Autodesk Inventor part; units mm, degrees
(part 3 of 3)
  line L1419 (-51.1011, -48.3705) -> (-50.3814, -49.0902) construction
  line L1420 (-50.3814, -49.0902) -> (-50.3814, -49.9795) construction
  spline S136 degree 3 poles (-46.3996, -18.0009) (-46.3996, -18.8902) (-47.1193, -19.6113) (-48.0086, -19.6113) knots 0 0 0 0 1 1 1 1
  line L1421 (-46.3996, -18.0009) -> (-46.3996, -18.8902) construction
  line L1422 (-46.3996, -18.8902) -> (-47.1193, -19.6113) construction
  line L1423 (-47.1193, -19.6113) -> (-48.0086, -19.6113) construction
  spline S137 degree 3 poles (-48.0086, -19.6113) (-48.8993, -19.6113) (-49.619, -18.8902) (-49.619, -18.0009) knots 0 0 0 0 1 1 1 1
  line L1424 (-48.0086, -19.6113) -> (-48.8993, -19.6113) construction
  line L1425 (-48.8993, -19.6113) -> (-49.619, -18.8902) construction
  line L1426 (-49.619, -18.8902) -> (-49.619, -18.0009) construction
  spline S138 degree 3 poles (-49.619, -18.0009) (-49.619, -17.1116) (-48.8993, -16.3919) (-48.0086, -16.3919) knots 0 0 0 0 1 1 1 1
  line L1427 (-49.619, -18.0009) -> (-49.619, -17.1116) construction
  line L1428 (-49.619, -17.1116) -> (-48.8993, -16.3919) construction
  line L1429 (-48.8993, -16.3919) -> (-48.0086, -16.3919) construction
  spline S139 degree 3 poles (-48.0086, -16.3919) (-47.1193, -16.3919) (-46.3996, -17.1116) (-46.3996, -18.0009) knots 0 0 0 0 1 1 1 1
  line L1430 (-48.0086, -16.3919) -> (-47.1193, -16.3919) construction
  line L1431 (-47.1193, -16.3919) -> (-46.3996, -17.1116) construction
  line L1432 (-46.3996, -17.1116) -> (-46.3996, -18.0009) construction
  spline S140 degree 3 poles (-72.7019, -7.3708) (-72.7019, -8.0905) (-73.2534, -8.6406) (-73.9731, -8.6406) knots 0 0 0 0 1 1 1 1
  line L1433 (-72.7019, -7.3708) -> (-72.7019, -8.0905) construction
  line L1434 (-72.7019, -8.0905) -> (-73.2534, -8.6406) construction
  line L1435 (-73.2534, -8.6406) -> (-73.9731, -8.6406) construction
  spline S141 degree 3 poles (-73.9731, -8.6406) (-74.6928, -8.6406) (-75.2429, -8.0905) (-75.2429, -7.3708) knots 0 0 0 0 1 1 1 1
  line L1436 (-73.9731, -8.6406) -> (-74.6928, -8.6406) construction
  line L1437 (-74.6928, -8.6406) -> (-75.2429, -8.0905) construction
  line L1438 (-75.2429, -8.0905) -> (-75.2429, -7.3708) construction
  spline S142 degree 3 poles (-75.2429, -7.3708) (-75.2429, -6.6497) (-74.6928, -6.0996) (-73.9731, -6.0996) knots 0 0 0 0 1 1 1 1
  line L1439 (-75.2429, -7.3708) -> (-75.2429, -6.6497) construction
  line L1440 (-75.2429, -6.6497) -> (-74.6928, -6.0996) construction
  line L1441 (-74.6928, -6.0996) -> (-73.9731, -6.0996) construction
  spline S143 degree 3 poles (-73.9731, -6.0996) (-73.2534, -6.0996) (-72.7019, -6.6497) (-72.7019, -7.3708) knots 0 0 0 0 1 1 1 1
  line L1442 (-73.9731, -6.0996) -> (-73.2534, -6.0996) construction
  line L1443 (-73.2534, -6.0996) -> (-72.7019, -6.6497) construction
  line L1444 (-72.7019, -6.6497) -> (-72.7019, -7.3708) construction
  spline S144 degree 3 poles (-72.7019, 7.3694) (-72.7019, 6.6497) (-73.2534, 6.0982) (-73.9731, 6.0982) knots 0 0 0 0 1 1 1 1
  line L1445 (-72.7019, 7.3694) -> (-72.7019, 6.6497) construction
  line L1446 (-72.7019, 6.6497) -> (-73.2534, 6.0982) construction
  line L1447 (-73.2534, 6.0982) -> (-73.9731, 6.0982) construction
  spline S145 degree 3 poles (-73.9731, 6.0982) (-74.6928, 6.0982) (-75.2429, 6.6497) (-75.2429, 7.3694) knots 0 0 0 0 1 1 1 1
  line L1448 (-73.9731, 6.0982) -> (-74.6928, 6.0982) construction
  line L1449 (-74.6928, 6.0982) -> (-75.2429, 6.6497) construction
  line L1450 (-75.2429, 6.6497) -> (-75.2429, 7.3694) construction
  spline S146 degree 3 poles (-75.2429, 7.3694) (-75.2429, 8.0891) (-74.6928, 8.6406) (-73.9731, 8.6406) knots 0 0 0 0 1 1 1 1
  line L1451 (-75.2429, 7.3694) -> (-75.2429, 8.0891) construction
  line L1452 (-75.2429, 8.0891) -> (-74.6928, 8.6406) construction
  line L1453 (-74.6928, 8.6406) -> (-73.9731, 8.6406) construction
  spline S147 degree 3 poles (-73.9731, 8.6406) (-73.2534, 8.6406) (-72.7019, 8.0891) (-72.7019, 7.3694) knots 0 0 0 0 1 1 1 1
  line L1454 (-73.9731, 8.6406) -> (-73.2534, 8.6406) construction
  line L1455 (-73.2534, 8.6406) -> (-72.7019, 8.0891) construction
  line L1456 (-72.7019, 8.0891) -> (-72.7019, 7.3694) construction
  spline S148 degree 3 poles (-46.3996, 18.0009) (-46.3996, 17.1116) (-47.1193, 16.3905) (-48.0086, 16.3905) knots 0 0 0 0 1 1 1 1
  line L1457 (-46.3996, 18.0009) -> (-46.3996, 17.1116) construction
  line L1458 (-46.3996, 17.1116) -> (-47.1193, 16.3905) construction
  line L1459 (-47.1193, 16.3905) -> (-48.0086, 16.3905) construction
  spline S149 degree 3 poles (-48.0086, 16.3905) (-48.8993, 16.3905) (-49.619, 17.1116) (-49.619, 18.0009) knots 0 0 0 0 1 1 1 1
  line L1460 (-48.0086, 16.3905) -> (-48.8993, 16.3905) construction
  line L1461 (-48.8993, 16.3905) -> (-49.619, 17.1116) construction
  line L1462 (-49.619, 17.1116) -> (-49.619, 18.0009) construction
  spline S150 degree 3 poles (-49.619, 18.0009) (-49.619, 18.8902) (-48.8993, 19.6099) (-48.0086, 19.6099) knots 0 0 0 0 1 1 1 1
  line L1463 (-49.619, 18.0009) -> (-49.619, 18.8902) construction
  line L1464 (-49.619, 18.8902) -> (-48.8993, 19.6099) construction
  line L1465 (-48.8993, 19.6099) -> (-48.0086, 19.6099) construction
  spline S151 degree 3 poles (-48.0086, 19.6099) (-47.1193, 19.6099) (-46.3996, 18.8902) (-46.3996, 18.0009) knots 0 0 0 0 1 1 1 1
  line L1466 (-48.0086, 19.6099) -> (-47.1193, 19.6099) construction
  line L1467 (-47.1193, 19.6099) -> (-46.3996, 18.8902) construction
  line L1468 (-46.3996, 18.8902) -> (-46.3996, 18.0009) construction
  spline S152 degree 3 poles (-50.3814, 50.0209) (-50.3814, 49.1316) (-51.1011, 48.4119) (-51.9904, 48.4119) knots 0 0 0 0 1 1 1 1
  line L1469 (-50.3814, 50.0209) -> (-50.3814, 49.1316) construction
  line L1470 (-50.3814, 49.1316) -> (-51.1011, 48.4119) construction
  line L1471 (-51.1011, 48.4119) -> (-51.9904, 48.4119) construction
  spline S153 degree 3 poles (-51.9904, 48.4119) (-52.8797, 48.4119) (-53.6008, 49.1316) (-53.6008, 50.0209) knots 0 0 0 0 1 1 1 1
  line L1472 (-51.9904, 48.4119) -> (-52.8797, 48.4119) construction
  line L1473 (-52.8797, 48.4119) -> (-53.6008, 49.1316) construction
  line L1474 (-53.6008, 49.1316) -> (-53.6008, 50.0209) construction
  spline S154 degree 3 poles (-53.6008, 50.0209) (-53.6008, 50.9102) (-52.8797, 51.6299) (-51.9904, 51.6299) knots 0 0 0 0 1 1 1 1
  line L1475 (-53.6008, 50.0209) -> (-53.6008, 50.9102) construction
  line L1476 (-53.6008, 50.9102) -> (-52.8797, 51.6299) construction
  line L1477 (-52.8797, 51.6299) -> (-51.9904, 51.6299) construction
  spline S155 degree 3 poles (-51.9904, 51.6299) (-51.1011, 51.6299) (-50.3814, 50.9102) (-50.3814, 50.0209) knots 0 0 0 0 1 1 1 1
  line L1478 (-51.9904, 51.6299) -> (-51.1011, 51.6299) construction
  line L1479 (-51.1011, 51.6299) -> (-50.3814, 50.9102) construction
  line L1480 (-50.3814, 50.9102) -> (-50.3814, 50.0209) construction
  spline S156 degree 3 poles (-7.7299, 44.0068) (-7.7299, 43.2871) (-8.2801, 42.7356) (-8.9998, 42.7356) knots 0 0 0 0 1 1 1 1
  line L1481 (-7.7299, 44.0068) -> (-7.7299, 43.2871) construction
  line L1482 (-7.7299, 43.2871) -> (-8.2801, 42.7356) construction
  line L1483 (-8.2801, 42.7356) -> (-8.9998, 42.7356) construction
  spline S157 degree 3 poles (-8.9998, 42.7356) (-9.7208, 42.7356) (-10.271, 43.2871) (-10.271, 44.0068) knots 0 0 0 0 1 1 1 1
  line L1484 (-8.9998, 42.7356) -> (-9.7208, 42.7356) construction
  line L1485 (-9.7208, 42.7356) -> (-10.271, 43.2871) construction
  line L1486 (-10.271, 43.2871) -> (-10.271, 44.0068) construction
  spline S158 degree 3 poles (-10.271, 44.0068) (-10.271, 44.7265) (-9.7208, 45.2766) (-8.9998, 45.2766) knots 0 0 0 0 1 1 1 1
  line L1487 (-10.271, 44.0068) -> (-10.271, 44.7265) construction
  line L1488 (-10.271, 44.7265) -> (-9.7208, 45.2766) construction
  line L1489 (-9.7208, 45.2766) -> (-8.9998, 45.2766) construction
  spline S159 degree 3 poles (-8.9998, 45.2766) (-8.2801, 45.2766) (-7.7299, 44.7265) (-7.7299, 44.0068) knots 0 0 0 0 1 1 1 1
  line L1490 (-8.9998, 45.2766) -> (-8.2801, 45.2766) construction
  line L1491 (-8.2801, 45.2766) -> (-7.7299, 44.7265) construction
  line L1492 (-7.7299, 44.7265) -> (-7.7299, 44.0068) construction
  spline S160 degree 3 poles (52.626, 50.0209) (52.626, 49.1316) (51.9063, 48.4119) (51.017, 48.4119) knots 0 0 0 0 1 1 1 1
  line L1493 (52.626, 50.0209) -> (52.626, 49.1316) construction
  line L1494 (52.626, 49.1316) -> (51.9063, 48.4119) construction
  line L1495 (51.9063, 48.4119) -> (51.017, 48.4119) construction
  spline S161 degree 3 poles (51.017, 48.4119) (50.1277, 48.4119) (49.408, 49.1316) (49.408, 50.0209) knots 0 0 0 0 1 1 1 1
  line L1496 (51.017, 48.4119) -> (50.1277, 48.4119) construction
  line L1497 (50.1277, 48.4119) -> (49.408, 49.1316) construction
  line L1498 (49.408, 49.1316) -> (49.408, 50.0209) construction
  spline S162 degree 3 poles (49.408, 50.0209) (49.408, 50.9102) (50.1277, 51.6299) (51.017, 51.6299) knots 0 0 0 0 1 1 1 1
  line L1499 (49.408, 50.0209) -> (49.408, 50.9102) construction
  line L1500 (49.408, 50.9102) -> (50.1277, 51.6299) construction
  line L1501 (50.1277, 51.6299) -> (51.017, 51.6299) construction
  spline S163 degree 3 poles (51.017, 51.6299) (51.9063, 51.6299) (52.626, 50.9102) (52.626, 50.0209) knots 0 0 0 0 1 1 1 1
  line L1502 (51.017, 51.6299) -> (51.9063, 51.6299) construction
  line L1503 (51.9063, 51.6299) -> (52.626, 50.9102) construction
  line L1504 (52.626, 50.9102) -> (52.626, 50.0209) construction
  spline S164 degree 3 poles (10.271, 44.0068) (10.271, 43.2871) (9.7208, 42.7356) (9.0011, 42.7356) knots 0 0 0 0 1 1 1 1
  line L1505 (10.271, 44.0068) -> (10.271, 43.2871) construction
  line L1506 (10.271, 43.2871) -> (9.7208, 42.7356) construction
  line L1507 (9.7208, 42.7356) -> (9.0011, 42.7356) construction
  spline S165 degree 3 poles (9.0011, 42.7356) (8.28, 42.7356) (7.7299, 43.2871) (7.7299, 44.0068) knots 0 0 0 0 1 1 1 1
  line L1508 (9.0011, 42.7356) -> (8.28, 42.7356) construction
  line L1509 (8.28, 42.7356) -> (7.7299, 43.2871) construction
  line L1510 (7.7299, 43.2871) -> (7.7299, 44.0068) construction
  spline S166 degree 3 poles (7.7299, 44.0068) (7.7299, 44.7265) (8.28, 45.2766) (9.0011, 45.2766) knots 0 0 0 0 1 1 1 1
  line L1511 (7.7299, 44.0068) -> (7.7299, 44.7265) construction
  line L1512 (7.7299, 44.7265) -> (8.28, 45.2766) construction
  line L1513 (8.28, 45.2766) -> (9.0011, 45.2766) construction
  spline S167 degree 3 poles (9.0011, 45.2766) (9.7208, 45.2766) (10.271, 44.7265) (10.271, 44.0068) knots 0 0 0 0 1 1 1 1
  line L1514 (9.0011, 45.2766) -> (9.7208, 45.2766) construction
  line L1515 (9.7208, 45.2766) -> (10.271, 44.7265) construction
  line L1516 (10.271, 44.7265) -> (10.271, 44.0068) construction
  spline S168 degree 3 poles (20.606, 18.0009) (20.606, 17.1116) (19.8863, 16.3905) (18.997, 16.3905) knots 0 0 0 0 1 1 1 1
  line L1517 (20.606, 18.0009) -> (20.606, 17.1116) construction
  line L1518 (20.606, 17.1116) -> (19.8863, 16.3905) construction
  line L1519 (19.8863, 16.3905) -> (18.997, 16.3905) construction
  spline S169 degree 3 poles (18.997, 16.3905) (18.1064, 16.3905) (17.3867, 17.1116) (17.3867, 18.0009) knots 0 0 0 0 1 1 1 1
  line L1520 (18.997, 16.3905) -> (18.1064, 16.3905) construction
  line L1521 (18.1064, 16.3905) -> (17.3867, 17.1116) construction
  line L1522 (17.3867, 17.1116) -> (17.3867, 18.0009) construction
  spline S170 degree 3 poles (17.3867, 18.0009) (17.3867, 18.8902) (18.1064, 19.6099) (18.997, 19.6099) knots 0 0 0 0 1 1 1 1
  line L1523 (17.3867, 18.0009) -> (17.3867, 18.8902) construction
  line L1524 (17.3867, 18.8902) -> (18.1064, 19.6099) construction
  line L1525 (18.1064, 19.6099) -> (18.997, 19.6099) construction
  spline S171 degree 3 poles (18.997, 19.6099) (19.8863, 19.6099) (20.606, 18.8902) (20.606, 18.0009) knots 0 0 0 0 1 1 1 1
  line L1526 (18.997, 19.6099) -> (19.8863, 19.6099) construction
  line L1527 (19.8863, 19.6099) -> (20.606, 18.8902) construction
  line L1528 (20.606, 18.8902) -> (20.606, 18.0009) construction
  spline S172 degree 3 poles (20.606, -18.0009) (20.606, -18.8902) (19.8863, -19.6113) (18.997, -19.6113) knots 0 0 0 0 1 1 1 1
  line L1529 (20.606, -18.0009) -> (20.606, -18.8902) construction
  line L1530 (20.606, -18.8902) -> (19.8863, -19.6113) construction
  line L1531 (19.8863, -19.6113) -> (18.997, -19.6113) construction
  spline S173 degree 3 poles (18.997, -19.6113) (18.1064, -19.6113) (17.3867, -18.8902) (17.3867, -18.0009) knots 0 0 0 0 1 1 1 1
  line L1532 (18.997, -19.6113) -> (18.1064, -19.6113) construction
  line L1533 (18.1064, -19.6113) -> (17.3867, -18.8902) construction
  line L1534 (17.3867, -18.8902) -> (17.3867, -18.0009) construction
  spline S174 degree 3 poles (17.3867, -18.0009) (17.3867, -17.1116) (18.1064, -16.3919) (18.997, -16.3919) knots 0 0 0 0 1 1 1 1
  line L1535 (17.3867, -18.0009) -> (17.3867, -17.1116) construction
  line L1536 (17.3867, -17.1116) -> (18.1064, -16.3919) construction
  line L1537 (18.1064, -16.3919) -> (18.997, -16.3919) construction
  spline S175 degree 3 poles (18.997, -16.3919) (19.8863, -16.3919) (20.606, -17.1116) (20.606, -18.0009) knots 0 0 0 0 1 1 1 1
  line L1538 (18.997, -16.3919) -> (19.8863, -16.3919) construction
  line L1539 (19.8863, -16.3919) -> (20.606, -17.1116) construction
  line L1540 (20.606, -17.1116) -> (20.606, -18.0009) construction
  spline S176 degree 3 poles (52.626, -49.9795) (52.626, -50.8688) (51.9063, -51.5885) (51.017, -51.5885) knots 0 0 0 0 1 1 1 1
  line L1541 (52.626, -49.9795) -> (52.626, -50.8688) construction
  line L1542 (52.626, -50.8688) -> (51.9063, -51.5885) construction
  line L1543 (51.9063, -51.5885) -> (51.017, -51.5885) construction
  spline S177 degree 3 poles (51.017, -51.5885) (50.1277, -51.5885) (49.408, -50.8688) (49.408, -49.9795) knots 0 0 0 0 1 1 1 1
  line L1544 (51.017, -51.5885) -> (50.1277, -51.5885) construction
  line L1545 (50.1277, -51.5885) -> (49.408, -50.8688) construction
  line L1546 (49.408, -50.8688) -> (49.408, -49.9795) construction
  spline S178 degree 3 poles (49.408, -49.9795) (49.408, -49.0902) (50.1277, -48.3705) (51.017, -48.3705) knots 0 0 0 0 1 1 1 1
  line L1547 (49.408, -49.9795) -> (49.408, -49.0902) construction
  line L1548 (49.408, -49.0902) -> (50.1277, -48.3705) construction
  line L1549 (50.1277, -48.3705) -> (51.017, -48.3705) construction
  spline S179 degree 3 poles (51.017, -48.3705) (51.9063, -48.3705) (52.626, -49.0902) (52.626, -49.9795) knots 0 0 0 0 1 1 1 1
  line L1550 (51.017, -48.3705) -> (51.9063, -48.3705) construction
  line L1551 (51.9063, -48.3705) -> (52.626, -49.0902) construction
  line L1552 (52.626, -49.0902) -> (52.626, -49.9795) construction
  spline S180 degree 3 poles (68.2982, 7.3694) (68.2982, 6.6497) (67.7467, 6.0982) (67.027, 6.0982) knots 0 0 0 0 1 1 1 1
  line L1553 (68.2982, 7.3694) -> (68.2982, 6.6497) construction
  line L1554 (68.2982, 6.6497) -> (67.7467, 6.0982) construction
  line L1555 (67.7467, 6.0982) -> (67.027, 6.0982) construction
  spline S181 degree 3 poles (67.027, 6.0982) (66.3073, 6.0982) (65.7558, 6.6497) (65.7558, 7.3694) knots 0 0 0 0 1 1 1 1
  line L1556 (67.027, 6.0982) -> (66.3073, 6.0982) construction
  line L1557 (66.3073, 6.0982) -> (65.7558, 6.6497) construction
  line L1558 (65.7558, 6.6497) -> (65.7558, 7.3694) construction
  spline S182 degree 3 poles (65.7558, 7.3694) (65.7558, 8.0891) (66.3073, 8.6406) (67.027, 8.6406) knots 0 0 0 0 1 1 1 1
  line L1559 (65.7558, 7.3694) -> (65.7558, 8.0891) construction
  line L1560 (65.7558, 8.0891) -> (66.3073, 8.6406) construction
  line L1561 (66.3073, 8.6406) -> (67.027, 8.6406) construction
  spline S183 degree 3 poles (67.027, 8.6406) (67.7467, 8.6406) (68.2982, 8.0891) (68.2982, 7.3694) knots 0 0 0 0 1 1 1 1
  line L1562 (67.027, 8.6406) -> (67.7467, 8.6406) construction
  line L1563 (67.7467, 8.6406) -> (68.2982, 8.0891) construction
  line L1564 (68.2982, 8.0891) -> (68.2982, 7.3694) construction
  spline S184 degree 3 poles (68.2982, -7.3708) (68.2982, -8.0905) (67.7467, -8.6406) (67.027, -8.6406) knots 0 0 0 0 1 1 1 1
  line L1565 (68.2982, -7.3708) -> (68.2982, -8.0905) construction
  line L1566 (68.2982, -8.0905) -> (67.7467, -8.6406) construction
  line L1567 (67.7467, -8.6406) -> (67.027, -8.6406) construction
  spline S185 degree 3 poles (67.027, -8.6406) (66.3073, -8.6406) (65.7558, -8.0905) (65.7558, -7.3708) knots 0 0 0 0 1 1 1 1
  line L1568 (67.027, -8.6406) -> (66.3073, -8.6406) construction
  line L1569 (66.3073, -8.6406) -> (65.7558, -8.0905) construction
  line L1570 (65.7558, -8.0905) -> (65.7558, -7.3708) construction
  spline S186 degree 3 poles (65.7558, -7.3708) (65.7558, -6.6497) (66.3073, -6.0996) (67.027, -6.0996) knots 0 0 0 0 1 1 1 1
  line L1571 (65.7558, -7.3708) -> (65.7558, -6.6497) construction
  line L1572 (65.7558, -6.6497) -> (66.3073, -6.0996) construction
  line L1573 (66.3073, -6.0996) -> (67.027, -6.0996) construction
  spline S187 degree 3 poles (67.027, -6.0996) (67.7467, -6.0996) (68.2982, -6.6497) (68.2982, -7.3708) knots 0 0 0 0 1 1 1 1
  line L1574 (67.027, -6.0996) -> (67.7467, -6.0996) construction
  line L1575 (67.7467, -6.0996) -> (68.2982, -6.6497) construction
  line L1576 (68.2982, -6.6497) -> (68.2982, -7.3708) construction
  spline S188 degree 3 poles (-25.3917, 18.0009) (-25.3917, 17.1116) (-26.1114, 16.3905) (-27.0006, 16.3905) knots 0 0 0 0 1 1 1 1
  line L1577 (-25.3917, 18.0009) -> (-25.3917, 17.1116) construction
  line L1578 (-25.3917, 17.1116) -> (-26.1114, 16.3905) construction
  line L1579 (-26.1114, 16.3905) -> (-27.0006, 16.3905) construction
  spline S189 degree 3 poles (-27.0006, 16.3905) (-27.8899, 16.3905) (-28.611, 17.1116) (-28.611, 18.0009) knots 0 0 0 0 1 1 1 1
  line L1580 (-27.0006, 16.3905) -> (-27.8899, 16.3905) construction
  line L1581 (-27.8899, 16.3905) -> (-28.611, 17.1116) construction
  line L1582 (-28.611, 17.1116) -> (-28.611, 18.0009) construction
  spline S190 degree 3 poles (-28.611, 18.0009) (-28.611, 18.8902) (-27.8899, 19.6099) (-27.0006, 19.6099) knots 0 0 0 0 1 1 1 1
  line L1583 (-28.611, 18.0009) -> (-28.611, 18.8902) construction
  line L1584 (-28.611, 18.8902) -> (-27.8899, 19.6099) construction
  line L1585 (-27.8899, 19.6099) -> (-27.0006, 19.6099) construction
  spline S191 degree 3 poles (-27.0006, 19.6099) (-26.1114, 19.6099) (-25.3917, 18.8902) (-25.3917, 18.0009) knots 0 0 0 0 1 1 1 1
  line L1586 (-27.0006, 19.6099) -> (-26.1114, 19.6099) construction
  line L1587 (-26.1114, 19.6099) -> (-25.3917, 18.8902) construction
  line L1588 (-25.3917, 18.8902) -> (-25.3917, 18.0009) construction
  spline S192 degree 3 poles (-25.3917, -18.0009) (-25.3917, -18.8902) (-26.1114, -19.6113) (-27.0006, -19.6113) knots 0 0 0 0 1 1 1 1
  line L1589 (-25.3917, -18.0009) -> (-25.3917, -18.8902) construction
  line L1590 (-25.3917, -18.8902) -> (-26.1114, -19.6113) construction
  line L1591 (-26.1114, -19.6113) -> (-27.0006, -19.6113) construction
  spline S193 degree 3 poles (-27.0006, -19.6113) (-27.8899, -19.6113) (-28.611, -18.8902) (-28.611, -18.0009) knots 0 0 0 0 1 1 1 1
  line L1592 (-27.0006, -19.6113) -> (-27.8899, -19.6113) construction
  line L1593 (-27.8899, -19.6113) -> (-28.611, -18.8902) construction
  line L1594 (-28.611, -18.8902) -> (-28.611, -18.0009) construction
  spline S194 degree 3 poles (-28.611, -18.0009) (-28.611, -17.1116) (-27.8899, -16.3919) (-27.0006, -16.3919) knots 0 0 0 0 1 1 1 1
  line L1595 (-28.611, -18.0009) -> (-28.611, -17.1116) construction
  line L1596 (-28.611, -17.1116) -> (-27.8899, -16.3919) construction
  line L1597 (-27.8899, -16.3919) -> (-27.0006, -16.3919) construction
  spline S195 degree 3 poles (-27.0006, -16.3919) (-26.1114, -16.3919) (-25.3917, -17.1116) (-25.3917, -18.0009) knots 0 0 0 0 1 1 1 1
  line L1598 (-27.0006, -16.3919) -> (-26.1114, -16.3919) construction
  line L1599 (-26.1114, -16.3919) -> (-25.3917, -17.1116) construction
  line L1600 (-25.3917, -17.1116) -> (-25.3917, -18.0009) construction
  line L1601 (-33.9895, 68.0217) -> (-25.0111, 68.0217)
  line L1602 (-25.0111, 50.0209) -> (-6.5015, 50.0209)
  line L1603 (6.5015, 50.0209) -> (25.0111, 50.0209)
  line L1604 (-6.5015, 50.0209) -> (-6.5015, 60.0168)
  line L1605 (-6.5015, 60.0168) -> (6.5015, 60.0168)
  line L1606 (6.5015, 60.0168) -> (6.5015, 50.0209)
  line L1607 (-25.0111, -67.9804) -> (-33.9895, -67.9804)
  line L1608 (-6.5015, -59.9754) -> (6.5015, -59.9754)
  line L1609 (6.5015, -59.9754) -> (6.5015, -49.9795)
  line L1610 (6.5015, -49.9795) -> (25.0111, -49.9795)
  line L1611 (-25.0111, -49.9795) -> (-6.5015, -49.9795)
  line L1612 (-6.5015, -49.9795) -> (-6.5015, -59.9754)
  line L1613 (-33.9895, 68.0217) -> (-36.9965, 66.4541)
  line L1614 (-36.9965, 66.4541) -> (-39.9195, 64.7183)
  line L1615 (-39.9195, 64.7183) -> (-42.7569, 62.897)
  line L1616 (-42.7569, 62.897) -> (-45.5103, 60.9488)
  line L1617 (-45.5103, 60.9488) -> (-48.1782, 58.8738)
  line L1618 (-48.1782, 58.8738) -> (-50.7206, 56.6705)
  line L1619 (-50.7206, 56.6705) -> (-53.2189, 54.3405)
  line L1620 (-53.2189, 54.3405) -> (-55.5903, 51.9263)
  line L1621 (-55.5903, 51.9263) -> (-57.8363, 49.428)
  line L1622 (-57.8363, 49.428) -> (-59.954, 46.8015)
  line L1623 (-59.954, 46.8015) -> (-61.9863, 44.0909)
  line L1624 (-61.9863, 44.0909) -> (-63.8917, 41.2962)
  line L1625 (-63.8917, 41.2962) -> (-65.6289, 38.3732)
  line L1626 (-65.6289, 38.3732) -> (-67.2807, 35.4503)
  line L1627 (-67.2807, 35.4503) -> (-68.7628, 32.4019)
  line L1628 (-68.7628, 32.4019) -> (-70.1609, 29.3094)
  line L1629 (-70.1609, 29.3094) -> (-71.3893, 26.1755)
  line L1630 (-71.3893, 26.1755) -> (-72.4482, 22.9561)
  line L1631 (-72.4482, 22.9561) -> (-73.3802, 19.6954)
  line L1632 (-73.3802, 19.6954) -> (-74.9892, 18.5083)
  line L1633 (-74.9892, 18.5083) -> (-76.4714, 17.153)
  line L1634 (-76.4714, 17.153) -> (-77.8267, 15.6708)
  line L1635 (-77.8267, 15.6708) -> (-79.0979, 14.1032)
  line L1636 (-79.0979, 14.1032) -> (-80.1995, 12.4101)
  line L1637 (-80.1995, 12.4101) -> (-81.1729, 10.6729)
  line L1638 (-81.1729, 10.6729) -> (-81.9781, 8.8515)
  line L1639 (-81.9781, 8.8515) -> (-82.6137, 6.9461)
  line L1640 (-82.6137, 6.9461) -> (-83.1211, 4.9979)
  line L1641 (-83.1211, 4.9979) -> (-83.4603, 3.007)
  line L1642 (-83.4603, 3.007) -> (-83.6298, 1.0161)
  line L1643 (-83.6298, 1.0161) -> (-83.6298, -0.9748)
  line L1644 (-83.6298, -0.9748) -> (-83.4603, -3.007)
  line L1645 (-83.4603, -3.007) -> (-83.1211, -4.9566)
  line L1646 (-83.1211, -4.9566) -> (-82.6137, -6.9048)
  line L1647 (-82.6137, -6.9048) -> (-81.9781, -8.8102)
  line L1648 (-81.9781, -8.8102) -> (-81.1729, -10.6315)
  line L1649 (-81.1729, -10.6315) -> (-80.1995, -12.4101)
  line L1650 (-80.1995, -12.4101) -> (-79.0979, -14.0618)
  line L1651 (-79.0979, -14.0618) -> (-77.8267, -15.6722)
  line L1652 (-77.8267, -15.6722) -> (-76.4714, -17.1116)
  line L1653 (-76.4714, -17.1116) -> (-74.9892, -18.4669)
  line L1654 (-74.9892, -18.4669) -> (-73.3802, -19.6954)
  line L1655 (-73.3802, -19.6954) -> (-72.4482, -22.9147)
  line L1656 (-72.4482, -22.9147) -> (-71.3466, -26.1341)
  line L1657 (-71.3466, -26.1341) -> (-70.1181, -29.268)
  line L1658 (-70.1181, -29.268) -> (-68.7628, -32.3591)
  line L1659 (-68.7628, -32.3591) -> (-67.2379, -35.4089)
  line L1660 (-67.2379, -35.4089) -> (-65.5862, -38.3319)
  line L1661 (-65.5862, -38.3319) -> (-63.8504, -41.2121)
  line L1662 (-63.8504, -41.2121) -> (-61.9436, -44.0068)
  line L1663 (-61.9436, -44.0068) -> (-59.9113, -46.7174)
  line L1664 (-59.9113, -46.7174) -> (-57.7935, -49.3439)
  line L1665 (-57.7935, -49.3439) -> (-55.5489, -51.8849)
  line L1666 (-55.5489, -51.8849) -> (-53.1761, -54.2991)
  line L1667 (-53.1761, -54.2991) -> (-50.7206, -56.5864)
  line L1668 (-50.7206, -56.5864) -> (-48.1368, -58.7897)
  line L1669 (-48.1368, -58.7897) -> (-45.4676, -60.9074)
  line L1670 (-45.4676, -60.9074) -> (-42.7142, -62.8556)
  line L1671 (-42.7142, -62.8556) -> (-39.8767, -64.6769)
  line L1672 (-39.8767, -64.6769) -> (-36.9965, -66.4128)
  line L1673 (-36.9965, -66.4128) -> (-33.9895, -67.9804)
  line L1674 (34.0322, -67.9804) -> (37.1248, -66.3287)
  line L1675 (37.1248, -66.3287) -> (40.1318, -64.5501)
  line L1676 (40.1318, -64.5501) -> (43.0547, -62.6433)
  line L1677 (43.0547, -62.6433) -> (45.9336, -60.611)
  line L1678 (45.9336, -60.611) -> (48.6456, -58.4078)
  line L1679 (48.6456, -58.4078) -> (51.3134, -56.1204)
  line L1680 (51.3134, -56.1204) -> (53.8545, -53.6649)
  line L1681 (53.8545, -53.6649) -> (56.2686, -51.1225)
  line L1682 (56.2686, -51.1225) -> (58.556, -48.4974)
  line L1683 (58.556, -48.4974) -> (60.7165, -45.744)
  line L1684 (60.7165, -45.744) -> (62.7915, -42.9065)
  line L1685 (62.7915, -42.9065) -> (64.6969, -39.9409)
  line L1686 (64.6969, -39.9409) -> (66.4769, -36.9338)
  line L1687 (66.4769, -36.9338) -> (68.0859, -33.8427)
  line L1688 (68.0859, -33.8427) -> (69.568, -30.666)
  line L1689 (69.568, -30.666) -> (70.9233, -27.4039)
  line L1690 (70.9233, -27.4039) -> (72.109, -24.1005)
  line L1691 (72.109, -24.1005) -> (73.1679, -20.7542)
  line L1692 (73.1679, -20.7542) -> (74.0158, -17.3653)
  line L1693 (74.0158, -17.3653) -> (74.7355, -13.935)
  line L1694 (74.7355, -13.935) -> (75.3284, -10.4619)
  line L1695 (75.3284, -10.4619) -> (75.7103, -6.9889)
  line L1696 (75.7103, -6.9889) -> (75.964, -3.5158)
  line L1697 (75.964, -3.5158) -> (76.0481, 0)
  line L1698 (76.0481, 0) -> (75.964, 3.5144)
  line L1699 (75.964, 3.5144) -> (75.7103, 7.0302)
  line L1700 (75.7103, 7.0302) -> (75.3284, 10.5033)
  line L1701 (75.3284, 10.5033) -> (74.7355, 13.9763)
  line L1702 (74.7355, 13.9763) -> (74.0158, 17.408)
  line L1703 (74.0158, 17.408) -> (73.1679, 20.7956)
  line L1704 (73.1679, 20.7956) -> (72.109, 24.1418)
  line L1705 (72.109, 24.1418) -> (70.9233, 27.4453)
  line L1706 (70.9233, 27.4453) -> (69.568, 30.6647)
  line L1707 (69.568, 30.6647) -> (68.0859, 33.8413)
  line L1708 (68.0859, 33.8413) -> (66.4769, 36.9338)
  line L1709 (66.4769, 36.9338) -> (64.6969, 39.9822)
  line L1710 (64.6969, 39.9822) -> (62.7915, 42.9052)
  line L1711 (62.7915, 42.9052) -> (60.7165, 45.7854)
  line L1712 (60.7165, 45.7854) -> (58.556, 48.496)
  line L1713 (58.556, 48.496) -> (56.2686, 51.1638)
  line L1714 (56.2686, 51.1638) -> (53.8545, 53.7062)
  line L1715 (53.8545, 53.7062) -> (51.3134, 56.1204)
  line L1716 (51.3134, 56.1204) -> (48.6456, 58.4491)
  line L1717 (48.6456, 58.4491) -> (45.9336, 60.6096)
  line L1718 (45.9336, 60.6096) -> (43.0547, 62.6846)
  line L1719 (43.0547, 62.6846) -> (40.1318, 64.5914)
  line L1720 (40.1318, 64.5914) -> (37.1248, 66.37)
  line L1721 (37.1248, 66.37) -> (34.0322, 68.0217)
  line L1722 (-25.0111, 50.0209) -> (-25.0111, 68.0217)
  line L1723 (25.0111, 50.0209) -> (25.0111, 68.0217)
  line L1724 (25.0111, 68.0217) -> (34.0322, 68.0217)
  line L1725 (-25.0111, -67.9804) -> (-25.0111, -49.9795)
  line L1726 (25.0111, -49.9795) -> (25.0111, -67.9804)
  line L1727 (25.0111, -67.9804) -> (34.0322, -67.9804)
  line L1728 (76.0481, 0) -> (-83.6298, 0)
  line L1729 (0, -67.9804) -> (0, 68.0217)
  point P0 (0, 0)
  point P1 (0, 0)
  point P2 (51.017, 50.0209)
  point P3 (51.017, -49.9795)
  point P4 (18.997, -18.0009)
  point P5 (18.997, 18.0009)
  point P6 (9.0011, 44.0068)
  point P7 (10.271, -44.0068)
  point P8 (9.0011, -44.0068)
  point P9 (-8.9998, 44.0068)
  point P10 (-8.9998, -44.0068)
  point P11 (67.027, 7.3694)
  point P12 (67.027, -7.3708)
  constraints: 2284 end point, 18 coincident, 4 point on line, 1 perpendicular, 588 other
sketch "Sketch3" plane through (0, 0, 0) normal (0, 1, 0) x (-1, 0, 0)
  line L0 (68.4126, 4.9694) -> (65.6413, 4.9694)
  line L1 (65.6413, 4.9694) -> (64.2557, 7.3694)
  line L2 (64.6021, 7.9694) -> (65.4681, 9.4694)
  line L3 (65.6413, 9.7694) -> (68.4126, 9.7694)
  line L4 (68.5858, 9.4694) -> (69.4519, 7.9694)
  line L5 (69.7983, 7.3694) -> (68.4126, 4.9694)
  line L6 (-75.3587, 4.9694) -> (-76.7444, 7.3694)
  line L7 (-76.7444, 7.3694) -> (-75.3587, 9.7694)
  line L8 (-75.3587, 9.7694) -> (-72.5875, 9.7694)
  line L9 (-72.5875, 9.7694) -> (-71.2018, 7.3694)
  line L10 (-71.2018, 7.3694) -> (-72.5875, 4.9694)
  line L11 (-72.5875, 4.9694) -> (-75.3587, 4.9694)
  line L12 (-75.3587, -9.7708) -> (-76.7444, -7.3708)
  line L13 (-76.7444, -7.3708) -> (-75.3587, -4.9708)
  line L14 (-75.3587, -4.9708) -> (-72.5875, -4.9708)
  line L15 (-72.5875, -4.9708) -> (-71.2018, -7.3708)
  line L16 (-71.2018, -7.3708) -> (-72.5875, -9.7708)
  line L17 (-72.5875, -9.7708) -> (-75.3587, -9.7708)
  line L18 (-72.5875, 9.7694) -> (-75.3587, 9.7694)
  line L19 (-75.3587, 9.7694) -> (-75.3587, 12.7694)
  line L20 (-75.3587, 12.7694) -> (-72.5875, 12.7694)
  line L21 (-72.5875, 12.7694) -> (-72.5875, 9.7694)
  line L22 (-71.2018, 7.3694) -> (-72.5875, 4.9694)
  line L23 (-72.5875, 4.9694) -> (-69.9894, 3.4694)
  line L24 (-69.9894, 3.4694) -> (-68.6037, 5.8694)
  line L25 (-68.6037, 5.8694) -> (-71.2018, 7.3694)
  line L26 (-75.3587, 4.9694) -> (-76.7444, 7.3694)
  line L27 (-76.7444, 7.3694) -> (-79.3425, 5.8694)
  line L28 (-79.3425, 5.8694) -> (-77.9568, 3.4694)
  line L29 (-77.9568, 3.4694) -> (-75.3587, 4.9694)
  line L30 (-72.5875, -9.7708) -> (-75.3587, -9.7708)
  line L31 (-75.3587, -9.7708) -> (-75.3587, -12.7708)
  line L32 (-75.3587, -12.7708) -> (-72.5875, -12.7708)
  line L33 (-72.5875, -12.7708) -> (-72.5875, -9.7708)
  line L34 (-76.7444, -7.3708) -> (-75.3587, -4.9708)
  line L35 (-75.3587, -4.9708) -> (-77.9568, -3.4708)
  line L36 (-77.9568, -3.4708) -> (-79.3425, -5.8708)
  line L37 (-79.3425, -5.8708) -> (-76.7444, -7.3708)
  line L38 (-71.2018, -7.3708) -> (-72.5875, -4.9708)
  line L39 (-72.5875, -4.9708) -> (-69.9894, -3.4708)
  line L40 (-69.9894, -3.4708) -> (-68.6037, -5.8708)
  line L41 (-68.6037, -5.8708) -> (-71.2018, -7.3708)
  line L42 (68.4126, 4.9694) -> (65.6413, 4.9694)
  line L43 (65.6413, 9.7694) -> (64.2557, 7.3694)
  line L44 (9.0011, 44.0068) -> (-8.9998, 44.0068)
  line L45 (-8.9998, 44.0068) -> (-8.9998, 39.7568)
  line L46 (-8.9998, 39.7568) -> (9.0011, 39.7568)
  line L47 (9.0011, 39.7568) -> (9.0011, 44.0068)
  line L48 (9.0011, 44.0068) -> (-8.9998, 44.0068)
  line L49 (9.0011, 48.2568) -> (9.0011, 44.0068)
  line L50 (9.0011, 44.0068) -> (7.5011, 44.0068)
  line L51 (7.5011, 44.0068) -> (7.5011, 48.3068)
  line L52 (7.5011, 48.3068) -> (9.0011, 48.3068)
  line L53 (9.0011, 48.3068) -> (9.0011, 44.0068)
  line L54 (7.5011, 48.3068) -> (17.5011, 48.3068)
  line L55 (17.5011, 48.3068) -> (17.5011, 50.3068)
  line L56 (17.5011, 50.3068) -> (7.5011, 50.3068)
  line L57 (7.5011, 50.3068) -> (7.5011, 48.3068)
  line L58 (-8.9998, 44.0068) -> (-7.4998, 44.0068)
  line L59 (-7.4998, 44.0068) -> (-7.4998, 48.3068)
  line L60 (-7.4998, 48.3068) -> (-8.9998, 48.3068)
  line L61 (-8.9998, 48.3068) -> (-8.9998, 44.0068)
  line L62 (-7.4998, 48.3068) -> (-17.4998, 48.3068)
  line L63 (-17.4998, 48.3068) -> (-17.4998, 50.3068)
  line L64 (-17.4998, 50.3068) -> (-7.4998, 50.3068)
  line L65 (-7.4998, 50.3068) -> (-7.4998, 48.3068)
  line L66 (68.759, 9.7694) -> (70.0983, 9.7694)
  line L67 (70.2983, 9.5694) -> (70.2983, 8.0694)
  line L68 (65.2949, 9.7694) -> (62.9557, 9.7694)
  line L69 (62.7557, 9.5694) -> (62.7557, 8.0694)
  line L70 (64.2557, 7.3694) -> (65.6413, 9.7694)
  line L71 (62.9557, 7.8694) -> (64.4289, 7.8694)
  line L72 (77.2983, 6.8694) -> (62.2983, 7.8694) construction
  line L73 (62.2983, 6.8694) -> (77.2983, 7.8694) construction
  arc A0 (68.759, 9.7694) -> (68.5858, 9.4694) centre (68.759, 9.5694) ccw
  arc A1 (70.2983, 9.5694) -> (70.0983, 9.7694) centre (70.0983, 9.5694) ccw
  arc A2 (70.0983, 7.8694) -> (70.2983, 8.0694) centre (70.0983, 8.0694) ccw
  arc A3 (65.4681, 9.4694) -> (65.2949, 9.7694) centre (65.2949, 9.5694) ccw
  arc A4 (62.9557, 9.7694) -> (62.7557, 9.5694) centre (62.9557, 9.5694) ccw
  arc A5 (62.7557, 8.0694) -> (62.9557, 7.8694) centre (62.9557, 8.0694) ccw
  arc A6 (64.4289, 7.8694) -> (64.6021, 7.9694) centre (64.4289, 8.0694) ccw
  line L74 (70.0983, 7.8694) -> (69.6251, 7.8694)
  arc A7 (69.4519, 7.9694) -> (69.6251, 7.8694) centre (69.6251, 8.0694) ccw
  line L75 (68.4126, 9.7694) -> (69.7983, 7.3694)
  line L76 (69.7983, 7.3694) -> (64.2557, 7.3694)
  line L77 (64.6021, 6.7694) -> (65.4681, 5.2694)
  line L78 (68.5858, 5.2694) -> (69.4519, 6.7694)
  line L79 (68.759, 4.9694) -> (70.0983, 4.9694)
  line L80 (70.2983, 5.1694) -> (70.2983, 6.6694)
  line L81 (65.2949, 4.9694) -> (62.9557, 4.9694)
  line L82 (62.7557, 5.1694) -> (62.7557, 6.6694)
  line L83 (62.9557, 6.8694) -> (64.4289, 6.8694)
  arc A8 (68.5858, 5.2694) -> (68.759, 4.9694) centre (68.759, 5.1694) ccw
  arc A9 (70.0983, 4.9694) -> (70.2983, 5.1694) centre (70.0983, 5.1694) ccw
  arc A10 (70.2983, 6.6694) -> (70.0983, 6.8694) centre (70.0983, 6.6694) ccw
  arc A11 (65.2949, 4.9694) -> (65.4681, 5.2694) centre (65.2949, 5.1694) ccw
  arc A12 (62.7557, 5.1694) -> (62.9557, 4.9694) centre (62.9557, 5.1694) ccw
  arc A13 (62.9557, 6.8694) -> (62.7557, 6.6694) centre (62.9557, 6.6694) ccw
  arc A14 (64.6021, 6.7694) -> (64.4289, 6.8694) centre (64.4289, 6.6694) ccw
  line L84 (70.0983, 6.8694) -> (69.6251, 6.8694)
  arc A15 (69.6251, 6.8694) -> (69.4519, 6.7694) centre (69.6251, 6.6694) ccw
  point P0 (0, 0)
  point P1 (67.027, 7.3694)
  point P2 (67.027, 7.3694)
  point P3 (9.0011, -44.0068)
  point P4 (-8.9998, -44.0068)
  point P5 (-73.9731, 7.3694)
  point P6 (-73.9731, -7.3708)
  point P7 (-73.9731, 7.3694)
  point P8 (-73.9731, -7.3708)
  point P9 (63.6073, 7.8694)
  point P10 (63.6073, 6.8694)
  dimension "d5" = 4.8
  dimension "d6" = 4.8
  dimension "d7" = 3
  dimension "d8" = 3
  dimension "d9" = 3
  dimension "d10" = 3
  dimension "d11" = 3
  dimension "d12" = 3
  dimension "d17" = 4.25
  dimension "d19" = 1.5
  dimension "d20" = 4.3
  dimension "d21" = 10
  dimension "d22" = 2
  dimension "d23" = 1.5
  dimension "d24" = 4.3
  dimension "d25" = 10
  dimension "d26" = 2
  dimension "d35" = 0.5
  dimension "d37" = 1.5
  dimension "d48" = 1
  dimension "d49" = 0.2
  dimension "d50" = 0.2
  dimension "d51" = 0.2
  constraints: 170 end point, 32 point on circle, 27 equal length, 25 symmetric about line, 17 point on line, 16 centre point, 16 tangent, 13 perpendicular, 10 horizontal, 5 equal radius, 2 midpoint, 1 coincident, 47 other
  measures "d5" distance between parallel lines of L6 L9
  measures "d6" distance between parallel lines of L12 L15
  measures "d7" distance of L18.end L19.end
  measures "d8" distance of L23.end L10.end
  measures "d9" distance of L27.end L26.end
  measures "d10" distance of L31.end L12.start
  measures "d11" distance of L35.end L13.end
  measures "d12" distance of L14.end L39.end
  measures "d17" distance of L45.end L44.end
  measures "d19" distance of L51.end L52.end
  measures "d20" distance of L50.end L51.end
  measures "d21" distance of L56.end L55.end
  measures "d22" distance of L55.end L54.end
  measures "d23" distance of L60.end L59.end
  measures "d24" distance of L59.end L58.end
  measures "d25" distance of L63.end L64.end
  measures "d26" distance of L62.end L63.end
  measures "d35" distance from line of L5.start L67
  measures "d37" distance from line of L1.end L69
  measures "d48" distance of L73.start L72.end
  measures "d49" radius of A0
  measures "d50" radius of A3
  measures "d51" radius of A7
extrude "Extrusion3" add sketch "Sketch3" along normal blind 2 contours L5 A15 L84 A10 L80 A9 L79 A8 | A11 L81 A12 L82 A13 L83 A14 L1 | L4 A0 L66 A1 L67 A2 L74 A7 | A6 L71 A5 L69 A4 L68 A3 L2
chamfer "Chamfer2" distance 0.2 angle 45 32 edges at (-70.2983, 2, 8.8194) (-70.2397, 2, 9.7108) (-69.4286, 2, 9.7694) (-68.5858, 2, 9.6694) (-69.0188, 2, 8.7194) (-69.5251, 2, 7.8962) (-69.8617, 2, 7.8694) (-70.2397, 2, 7.928) (-69.0188, 2, 6.0194) (-68.5858, 2, 5.0694) (-69.4286, 2, 4.9694) (-70.2397, 2, 5.028) (-70.2983, 2, 5.9194) (-70.2397, 2, 6.8108) (-69.8617, 2, 6.8694) (-69.5251, 2, 6.8426) (-65.0351, 2, 6.0194) (-64.5289, 2, 6.8426) (-63.6923, 2, 6.8694) (-62.8143, 2, 6.8108) (-62.7557, 2, 5.9194) (-62.8143, 2, 5.028) (-64.1253, 2, 4.9694) (-65.4681, 2, 5.0694) (-63.6923, 2, 7.8694) (-64.5289, 2, 7.8962) (-65.0351, 2, 8.7194) (-65.4681, 2, 9.6694) (-64.1253, 2, 9.7694) (-62.8143, 2, 9.7108) (-62.7557, 2, 8.8194) (-62.8143, 2, 7.928)
sketch "Sketch5" plane through (0, 0, 0) normal (0, -1, 0) x (1, 0, 0)
  line L0 (-65.2949, 9.7694) -> (-62.9557, 9.7694) projected
  arc A0 (-65.2949, 9.7694) -> (-65.4681, 9.4694) centre (-65.2949, 9.5694) ccw projected
  line L1 (-64.6021, 7.9694) -> (-65.4681, 9.4694) projected
  arc A1 (-64.6021, 7.9694) -> (-64.4289, 7.8694) centre (-64.4289, 8.0694) ccw projected
  line L2 (-62.9557, 7.8694) -> (-64.4289, 7.8694) projected
  arc A2 (-62.9557, 7.8694) -> (-62.7557, 8.0694) centre (-62.9557, 8.0694) ccw projected
  line L3 (-62.7557, 9.5694) -> (-62.7557, 8.0694) projected
  arc A3 (-62.7557, 9.5694) -> (-62.9557, 9.7694) centre (-62.9557, 9.5694) ccw projected
  line L4 (-76.0481, 0) -> (83.6298, 0) projected
  line L5 (-70.2983, 11.7694) -> (-52.7557, 11.7694)
  line L6 (-52.7557, 11.7694) -> (-52.7557, 0)
  line L7 (-52.7557, 0) -> (-70.2983, 0)
  line L8 (-70.2983, 0) -> (-70.2983, 11.7694)
  line L9 (-70.2983, 8.0694) -> (-70.2983, 9.5694) projected
  point P0 (0, 0)
  dimension "d60" = 10
  dimension "d74" = 0
  dimension "d75" = 2
  constraints: 8 end point, 2 parallel, 1 horizontal, 1 perpendicular, 1 point on line
  measures "d60" distance between parallel lines of L6 L3
  measures "d74" distance between parallel lines of L9 L8
  measures "d75" distance between parallel lines of L0 L5
extrude "Extrusion4" add sketch "Sketch5" along normal blind 5 contours L0 A3 L3 A2 L2 A1 L1 A0 | L8 L5 L6 L4
sketch "Sketch7" plane through (0, 0, 0) normal (0, 1, 0) x (1, 0, 0)
  line L0 (-62.7557, -6.6694) -> (-62.7557, -5.1694) projected
  line L1 (-64.4289, -6.8694) -> (-62.9557, -6.8694) projected
  point P0 (0, 0)
  point P1 (-58.7557, -6.8694)
  point P2 (-67.027, -7.3694)
  dimension "d65" = 4
  dimension "d66" = 0
  measures "d65" distance from line of point (-58.756, -6.869) L0
  measures "d66" distance from line of L1 point (-58.756, -6.869)
hole "Hole1" at (-58.7557, 0, 6.8694) direction (0, -1, 0) diameter 3.2 end through all counterbore diameter 6 counterbore depth 3.5
hole "Hole3" at (72.7019, 0, 7.3694) at (73.9731, 0, 8.6406) at (-67.027, 0, 7.3694) direction (0, -1, 0) diameter 3 end through all
mirror "Mirror1" about plane through (-70.2983, 0, 0) normal (0, 0, -1) of "Extrusion4", "Hole1", "Extrusion3", "Chamfer2", "Hole3"
body "Solid3"
